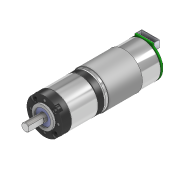
# Autodesk Inventor part: motor-ch-36gp-555
Saved by Autodesk Inventor 2020 (Build 240168000, 168)
## iProperties
Created: 2019-12-06
Part Number: motor-ch-36gp-555
Material: Generic
Document SubType Name: Modeling
Designer: Aespen-CAD
Density: 1 g/cm^3
Appearance: Default
Author: Aespen-CAD
Autodesk Inventor part; units mm, degrees
sketch "Sketch1" plane through (0, 0, 0) normal (0, 0, 1) x (1, 0, 0)
  circle A0 centre (0, 0) radius 18
  dimension "d0" = 36
  constraints: 1 centre point, 1 coincident
  measures "d0" diameter of A0
extrude "Extrusion1" add sketch "Sketch1" along normal blind 57
fillet "Fillet1" radius 1.5 1 edges at (-18, 0, 57)
sketch "Sketch2" plane through (0, 0, 57) normal (0, 0, 1) x (1, 0, 0)
  circle A0 centre (0, 0) radius 18
  constraints: 1 centre point, 1 coincident
extrude "Extrusion2" add sketch "Sketch2" along normal blind 6
fillet "Fillet2" radius 0.4 1 edges at (-18, 0, 63)
sketch "Sketch3" plane through (0, 0, 63) normal (0, 0, 1) x (1, 0, 0)
  circle A0 centre (0, 0) radius 18
  dimension "d7" = 36
  constraints: 1 centre point, 1 coincident
  measures "d7" diameter of A0
extrude "Extrusion3" add sketch "Sketch3" along normal blind 27.5
chamfer "Chamfer1" distance 0.4 angle 45 2 edges at (-18, 0, 90.5) (-18, 0, 63)
sketch "Sketch4" plane through (0, 0, 90.5) normal (0, 0, 1) x (1, 0, 0)
  circle A0 centre (0, 0) radius 18
  dimension "d13" = 36
  constraints: 1 centre point, 1 coincident
  measures "d13" diameter of A0
extrude "Extrusion4" add sketch "Sketch4" along normal blind 9
sketch "Sketch5" plane through (0, 0, 99.5) normal (0, 0, 1) x (1, 0, 0)
  circle A0 centre (0, 0) radius 11
  circle A1 centre (0, 0) radius 8.1
  dimension "d16" = 22
  dimension "d17" = 16.2
  constraints: 2 centre point, 2 coincident
  measures "d16" diameter of A0
  measures "d17" diameter of A1
extrude "Extrusion5" add sketch "Sketch5" along normal blind 2
sketch "Sketch6" plane through (0, 0, 99.5) normal (0, 0, 1) x (1, 0, 0)
  circle A0 centre (0, 0) radius 8
  circle A1 centre (0, 0) radius 4.1
  dimension "d20" = 16
  dimension "d21" = 8.2
  constraints: 2 centre point, 2 coincident
  measures "d20" diameter of A0
  measures "d21" diameter of A1
extrude "Extrusion6" add sketch "Sketch6" along normal blind 1
sketch "Sketch7" plane through (0, 0, 99.5) normal (0, 0, 1) x (1, 0, 0)
  circle A0 centre (0, 0) radius 4
  dimension "d24" = 8
  constraints: 1 centre point, 1 coincident
  measures "d24" diameter of A0
extrude "Extrusion7" add sketch "Sketch7" along normal blind 19.5
sketch "Sketch8" plane through (0, 0, 119) normal (0, 0, 1) x (1, 0, 0)
  line L0 (3, 5.7758) -> (10.3081, 5.7758)
  line L1 (10.3081, 5.7758) -> (10.3081, -11.4337)
  line L2 (10.3081, -11.4337) -> (3, -11.4337)
  line L3 (3, -11.4337) -> (3, 5.7758)
  point P0 (0, 0)
  dimension "d27" = 3
  constraints: 8 end point, 2 parallel, 1 horizontal, 1 perpendicular
  measures "d27" distance from line of L3 point (0, 0)
extrude "Extrusion8" cut sketch "Sketch8" against normal blind 15
chamfer "Chamfer2" distance 0.4 angle 45 1 edges at (-4, 0, 119)
sketch "Sketch9" plane through (0, 0, 0) normal (0, 0, -1) x (-1, 0, 0)
  line L0 (-14.5, 2) -> (-14, 2)
  line L1 (-14, 2) -> (-14, -2)
  line L2 (-14, -2) -> (-14.5, -2)
  line L3 (-14.5, -2) -> (-14.5, 2)
  line L4 (14, 2) -> (14.5, 2)
  line L5 (14.5, 2) -> (14.5, -2)
  line L6 (14.5, -2) -> (14, -2)
  line L7 (14, -2) -> (14, 2)
  point P0 (0, 0)
  dimension "d33" = 0.5
  dimension "d34" = 4
  dimension "d35" = 0.5
  dimension "d36" = 4
  dimension "d37" = 28
  dimension "d38" = 14
  dimension "d39" = 2
  dimension "d40" = 2
  constraints: 16 end point, 4 parallel, 2 horizontal, 2 perpendicular
  measures "d33" distance of L1.end L2.end
  measures "d34" distance of L0.end L1.end
  measures "d35" distance of L5.end L6.end
  measures "d36" distance of L4.end L5.end
  measures "d37" distance between parallel lines of L7 L1
  measures "d38" distance from line of point (0, 0) L7
  measures "d39" vertical distance of point (0, 0) L0.start
  measures "d40" distance from line of point (0, 0) L4
extrude "Extrusion9" add sketch "Sketch9" along normal blind 6
chamfer "Chamfer3" distance 0.8 angle 45 4 edges at (14.25, 2, -6) (14.25, -2, -6) (-14.25, 2, -6) (-14.25, -2, -6)
sketch "Sketch10" plane through (0, 0, 0) normal (0, 0, -1) x (-1, 0, 0)
  circle A0 centre (0, 0) radius 5
  circle A1 centre (0, 0) radius 1.6
  dimension "d46" = 10
  dimension "d47" = 3.2
  constraints: 2 centre point, 2 coincident
  measures "d46" diameter of A0
  measures "d47" diameter of A1
extrude "Extrusion10" add sketch "Sketch10" along normal blind 2.5
sketch "Sketch11" plane through (0, 0, -2.5) normal (0, 0, -1) x (-1, 0, 0)
  circle A0 centre (0, 0) radius 3.5
  arc A1 (-3, -1.99) -> (-3, 1.99) centre (0, 0) ccw projected
  circle A2 centre (0, 0) radius 1.6
  dimension "d50" = 7
  constraints: 2 centre point, 2 coincident
  measures "d50" diameter of A0
extrude "Extrusion11" add sketch "Sketch11" along normal blind 1.5
fillet "Fillet3" radius 0.4 2 edges at (3.5, 0, -4) (5, 0, -2.5)
sketch "Sketch13" plane through (0, 0, 0) normal (0, 0, -1) x (-1, 0, 0)
  circle A0 centre (0, 0) radius 1.5
  dimension "d54" = 3
  constraints: 1 centre point, 1 coincident
  measures "d54" diameter of A0
extrude "Extrusion12" add sketch "Sketch13" along normal blind 12
sketch "Sketch14" plane through (0, 0, -2.5) normal (0, 0, -1) x (-1, 0, 0)
  circle A0 centre (0, 0) radius 4 projected
  circle A1 centre (0, 0) radius 18
  line L0 (-14.75, 2.5248) -> (-13.75, 2.5248)
  line L1 (-13.75, 2.5248) -> (-13.75, -2.4752)
  line L2 (-13.75, -2.4752) -> (-14.75, -2.4752)
  line L3 (-14.75, -2.4752) -> (-14.75, 2.5248)
  line L4 (13.75, 2.5248) -> (14.75, 2.5248)
  line L5 (14.75, 2.5248) -> (14.75, -2.4752)
  line L6 (14.75, -2.4752) -> (13.75, -2.4752)
  line L7 (13.75, -2.4752) -> (13.75, 2.5248)
  circle A2 centre (0, 0) radius 5 projected
  circle A3 centre (0, 0) radius 5.5
  line L8 (-9, 18) -> (9, 18)
  line L9 (9, 18) -> (9, 14.9704)
  line L10 (9, 14.9704) -> (-9, 14.9704)
  line L11 (-9, 14.9704) -> (-9, 18)
  point P0 (-9, 15.5885)
  point P1 (0, 18)
  point P2 (9, 15.5885)
  dimension "d57" = 1
  dimension "d58" = 5
  dimension "d59" = 5
  dimension "d60" = 1
  dimension "d61" = 27.5
  dimension "d62" = 13.75
  dimension "d63" = 11
  dimension "d66" = 18
  dimension "d67" = 36
  dimension "d68" = 9
  constraints: 24 end point, 6 parallel, 3 horizontal, 3 perpendicular, 2 centre point, 2 coincident, 1 point on line, 1 tangent
  measures "d57" distance of L5.end L6.end
  measures "d58" distance of L4.end L5.end
  measures "d59" distance of L0.end L1.end
  measures "d60" distance of L0.start L0.end
  measures "d61" distance between parallel lines of L7 L1
  measures "d62" distance from line of A2.centre L1
  measures "d63" diameter of A3
  measures "d66" distance of L9.end L10.end
  measures "d67" diameter of A1
  measures "d68" distance from line of L11 point (0, 0)
extrude "Extrusion13" add sketch "Sketch14" against normal blind 1.6 contours A1 L11 L10 L9 | L9 L10 L11 A1 | A1 L8 L9 | L11 L8 A1
ref_plane "Work Plane1" through (0, 0, -5) normal (0, 0, -1) x (-1, 0, 0)
sketch "Sketch15" plane through (0, 0, -5) normal (0, 0, -1) x (-1, 0, 0)
  circle A0 centre (0, 0) radius 1.5 projected
  circle A1 centre (0, 0) radius 1.6
  circle A2 centre (0, 0) radius 9
  dimension "d70" = 3.2
  dimension "d71" = 18
  constraints: 2 centre point, 2 coincident
  measures "d70" diameter of A1
  measures "d71" diameter of A2
extrude "Extrusion14" add sketch "Sketch15" along normal blind 3 contours A2
sketch "Sketch16" plane through (0, 0, -8) normal (0, 0, -1) x (-1, 0, 0)
  circle A0 centre (0, 0) radius 9 projected
  circle A1 centre (0, 0) radius 7.5
  circle A2 centre (0, 0) radius 1.6
  dimension "d74" = 15
  dimension "d75" = 3.2
  constraints: 2 centre point, 2 coincident
  measures "d74" diameter of A1
  measures "d75" diameter of A2
extrude "Extrusion15" cut sketch "Sketch16" against normal blind 1.5 contours A1
fillet "Fillet4" radius 0.6 2 edges at (7.5, 0, -8) (7.5, 0, -6.5)
sketch "Sketch17" plane through (0, 0, 99.5) normal (0, 0, 1) x (1, 0, 0)
  circle A0 centre (0, 0) radius 1.5 construction
  line L0 (0, 0) -> (32.3265, 32.3265) construction
  line L1 (0, 0) -> (45.7166, 0) construction
  circle A1 centre (10.253, 10.253) radius 3
  line L2 (8.1317, 12.3744) -> (12.3744, 8.1317)
  line L3 (12.3744, 8.1317) -> (17.0459, 12.8033)
  line L4 (17.0459, 12.8033) -> (12.8033, 17.0459)
  line L5 (12.8033, 17.0459) -> (8.1317, 12.3744)
  circle A2 centre (-10.253, 10.253) radius 3
  line L6 (-8.1317, 12.3744) -> (-12.8033, 17.0459)
  line L7 (-12.8033, 17.0459) -> (-17.0459, 12.8033)
  line L8 (-17.0459, 12.8033) -> (-12.3744, 8.1317)
  line L9 (-12.3744, 8.1317) -> (-8.1317, 12.3744)
  circle A3 centre (-10.253, -10.253) radius 3
  line L10 (-12.3744, -8.1317) -> (-17.0459, -12.8033)
  line L11 (-17.0459, -12.8033) -> (-12.8033, -17.0459)
  line L12 (-12.8033, -17.0459) -> (-8.1317, -12.3744)
  line L13 (-8.1317, -12.3744) -> (-12.3744, -8.1317)
  circle A4 centre (10.253, -10.253) radius 3
  line L14 (8.1317, -12.3744) -> (12.8033, -17.0459)
  line L15 (12.8033, -17.0459) -> (17.0459, -12.8033)
  line L16 (17.0459, -12.8033) -> (12.3744, -8.1317)
  line L17 (12.3744, -8.1317) -> (8.1317, -12.3744)
  dimension "d79" = 45
  dimension "d80" = 6
  dimension "d81" = 14.5
  dimension "d84" = 360
  constraints: 36 end point, 8 point on circle, 4 centre point, 2 parallel, 1 equal length, 1 horizontal, 1 perpendicular, 1 point on line, 1 tangent, 41 other
  measures "d79" angle of L1 L0
  measures "d80" diameter of A1
  measures "d81" distance of point (0, 0) A1.centre
extrude "Extrusion16" cut sketch "Sketch17" against normal blind 4
sketch "Sketch18" plane through (0, 0, 95.5) normal (0, 0, 1) x (1, 0, 0)
  arc A0 (8.1317, 12.3744) -> (12.3744, 8.1317) centre (10.253, 10.253) ccw projected
  circle A1 centre (10.253, 10.253) radius 2.8
  line L0 (11.8809, 10.8447) -> (11.5793, 9.1391)
  line L1 (11.5793, 9.1391) -> (9.9515, 8.5475)
  line L2 (9.9515, 8.5475) -> (8.6252, 9.6614)
  line L3 (8.6252, 9.6614) -> (8.9267, 11.367)
  line L4 (8.9267, 11.367) -> (10.5546, 11.9586)
  line L5 (10.5546, 11.9586) -> (11.8809, 10.8447)
  circle A2 centre (0, 0) radius 1.6 projected
  circle A3 centre (-10.253, 10.253) radius 2.8
  line L6 (-10.8447, 11.8809) -> (-9.1391, 11.5793)
  line L7 (-9.1391, 11.5793) -> (-8.5475, 9.9515)
  line L8 (-8.5475, 9.9515) -> (-9.6614, 8.6252)
  line L9 (-9.6614, 8.6252) -> (-11.367, 8.9267)
  line L10 (-11.367, 8.9267) -> (-11.9586, 10.5546)
  line L11 (-11.9586, 10.5546) -> (-10.8447, 11.8809)
  circle A4 centre (-10.253, -10.253) radius 2.8
  line L12 (-11.8809, -10.8447) -> (-11.5793, -9.1391)
  line L13 (-11.5793, -9.1391) -> (-9.9515, -8.5475)
  line L14 (-9.9515, -8.5475) -> (-8.6252, -9.6614)
  line L15 (-8.6252, -9.6614) -> (-8.9267, -11.367)
  line L16 (-8.9267, -11.367) -> (-10.5546, -11.9586)
  line L17 (-10.5546, -11.9586) -> (-11.8809, -10.8447)
  circle A5 centre (10.253, -10.253) radius 2.8
  line L18 (10.8447, -11.8809) -> (9.1391, -11.5793)
  line L19 (9.1391, -11.5793) -> (8.5475, -9.9515)
  line L20 (8.5475, -9.9515) -> (9.6614, -8.6252)
  line L21 (9.6614, -8.6252) -> (11.367, -8.9267)
  line L22 (11.367, -8.9267) -> (11.9586, -10.5546)
  line L23 (11.9586, -10.5546) -> (10.8447, -11.8809)
  dimension "d88" = 5.6
  dimension "d89" = 3
  dimension "d90" = 14.5
  dimension "d93" = 360
  constraints: 48 end point, 4 centre point, 2 coincident, 74 other
  measures "d88" diameter of A1
  measures "d89" distance between parallel lines of L2 L5
  measures "d90" distance of A1.centre A2.centre
extrude "Extrusion17" add sketch "Sketch18" along normal blind 3 contours A1 | A3 | A4 | A5
sketch "Sketch19" plane through (0, 0, 99.5) normal (0, 0, 1) x (1, 0, 0)
  circle A0 centre (0, 14) radius 1.5
  circle A1 centre (-14, 0) radius 1.5
  circle A2 centre (0, -14) radius 1.5
  circle A3 centre (14, 0) radius 1.5
  point P0 (0, 0)
  dimension "d97" = 3
  dimension "d98" = 14
  dimension "d101" = 360
  constraints: 4 centre point, 9 other
  measures "d97" diameter of A0
  measures "d98" distance of point (0, 0) A0.centre
hole "Hole1" at (-14, 0, 99.5) at (0, 14, 99.5) at (14, 0, 99.5) at (0, -14, 99.5) direction (0, 0, -1) diameter 2.459 depth 8 thread size "M3x0.5" class "6H" standard "ANSI Metric M Profile"
ref_plane "Work Plane2" through (0, 0, -2.55) normal (0, 0, -1) x (-1, 0, 0)
sketch "Sketch20" plane through (0, 0, -2.55) normal (0, 0, -1) x (-1, 0, 0)
  line L0 (-9, 18) -> (9, 18) projected
  line L1 (-9, 18) -> (9, 18)
  line L2 (9, 18) -> (9, 11)
  line L3 (9, 11) -> (-9, 11)
  line L4 (-9, 11) -> (-9, 18)
  point P0 (0, 0)
  dimension "d104" = 18
  dimension "d105" = 7
  constraints: 8 end point, 2 parallel, 1 horizontal, 1 perpendicular
  measures "d104" distance of L2.end L3.end
  measures "d105" distance of L1.end L2.end
extrude "Extrusion18" add sketch "Sketch20" along normal blind 5.5
sketch "Sketch21" plane through (-9, 18, -2.55) normal (0, 1, 0) x (1, 0, 0)
  line L0 (0.5, 5) -> (17.5, 5)
  line L1 (17.5, 5) -> (17.5, 0.5)
  line L2 (17.5, 0.5) -> (0.5, 0.5)
  line L3 (0.5, 0.5) -> (0.5, 5)
  line L4 (18, 0) -> (18, 5.5) projected
  line L5 (0, 5.5) -> (18, 5.5) projected
  point P0 (9, -2.55)
  dimension "d108" = 17
  dimension "d109" = 4.5
  dimension "d110" = 0.5
  dimension "d111" = 0.5
  constraints: 8 end point, 2 parallel, 1 horizontal, 1 perpendicular
  measures "d108" distance of L1.end L2.end
  measures "d109" distance of L0.end L1.end
  measures "d110" distance between parallel lines of L4 L1
  measures "d111" distance between parallel lines of L5 L0
extrude "Extrusion19" cut sketch "Sketch21" against normal blind 5
ref_plane "Work Plane3" through (0, 0, 53) normal (0, 0, -1) x (-1, 0, 0)
sketch "Sketch22" plane through (0, 0, 53) normal (0, 0, -1) x (-1, 0, 0)
  circle A0 centre (0, 0) radius 18.01
  circle A1 centre (0, 0) radius 18.7
  line L0 (3.5, -21.754) -> (-3.5, -21.754)
  line L1 (-3.5, -21.754) -> (-3.5, -13.1412)
  line L2 (-3.5, -13.1412) -> (3.5, -13.1412)
  line L3 (3.5, -13.1412) -> (3.5, -21.754)
  point P0 (3.5, -17.6666)
  point P1 (3.5, -18.3695)
  point P2 (-3.5, -18.3695)
  point P3 (-3.5, -17.6666)
  dimension "d122" = 36.02
  dimension "d123" = 37.4
  dimension "d124" = 7
  dimension "d125" = 3.5
  constraints: 8 end point, 2 centre point, 2 coincident, 2 parallel, 1 horizontal, 1 perpendicular
  measures "d122" diameter of A0
  measures "d123" diameter of A1
  measures "d124" distance of L1.end L2.end
  measures "d125" distance from line of point (0, 0) L3
extrude "Extrusion20" add sketch "Sketch22" along normal blind 34 contours A0 L1 A1 L3 picked at (18.1253, 2.884)
equation "\"d39\" = 0.5 * d34"
equation "\"d62\" = 0.5 * d61"
body "Solid1"
